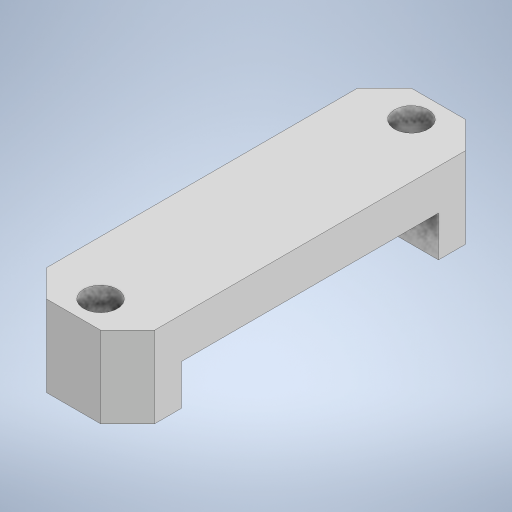
# Autodesk Inventor part: 스텝모터 드라이버 홀더
Saved by Autodesk Inventor 2023 (Build 270158000, 158)
## iProperties
Created: 2022-11-11
Part Number: 스텝모터 드라이버 홀더
Material: 일반
Document SubType Name: Modeling
Designer: hyunsu
Density: 1 g/cm^3
Appearance: 기본값
Author: hyunsu
Autodesk Inventor part; units mm, degrees
ref_plane "YZ Plane" through (0, 0, 0) normal (1, 0, 0) x (0, 1, 0)
ref_plane "XZ Plane" through (0, 0, 0) normal (0, 1, 0) x (-1, 0, 0)
ref_plane "XY Plane" through (0, 0, 0) normal (0, 0, 1) x (1, 0, 0)
sketch "스케치1" plane through (0, 0, 0) normal (0, 1, 0) x (-1, 0, 0)
  line L0 (4, 13.5) -> (-4, 13.5)
  line L1 (-4, 13.5) -> (-4, -13.5)
  line L2 (-4, -13.5) -> (4, -13.5)
  line L3 (4, -13.5) -> (4, 13.5)
  line L4 (4, 13.5) -> (-4, -13.5) construction
  line L5 (-4, 13.5) -> (4, -13.5) construction
  line L6 (4, 9.5) -> (-4, 9.5)
  line L7 (0, 0) -> (3.2228, 0)
  line L8 (4, -9.5) -> (-4, -9.5)
  circle A0 centre (0, 11.5) radius 1.25
  circle A1 centre (0, -11.5) radius 1.25
  point P0 (-4, -9.5)
  dimension "d0" = 8
  dimension "d1" = 27
  dimension "d2" = 4
  dimension "d3" = 2.5
  dimension "d4" = 2
  constraints: 18 end point, 3 symmetric about line, 2 centre point, 2 horizontal, 2 midpoint, 2 parallel, 2 perpendicular, 2 point on line, 1 vertical alignment, 1 other
  measures "d0" distance of L1.end L2.end
  measures "d1" distance of L0.end L1.end
  measures "d2" distance between parallel lines of L0 L6
  measures "d3" diameter of A0
  measures "d4" distance from line of L0 A0.centre
extrude "돌출1" add sketch "스케치1" against normal blind 3 contours L3 L6 L1 L0 | L3 L2 L1 L8
extrude "돌출2" add sketch "스케치1" along normal blind 3
chamfer "모따기1" distance 2 angle 45 4 edges at (4, 0, -13.5) (4, 0, 13.5) (-4, 0, 13.5) (-4, 0, -13.5)
